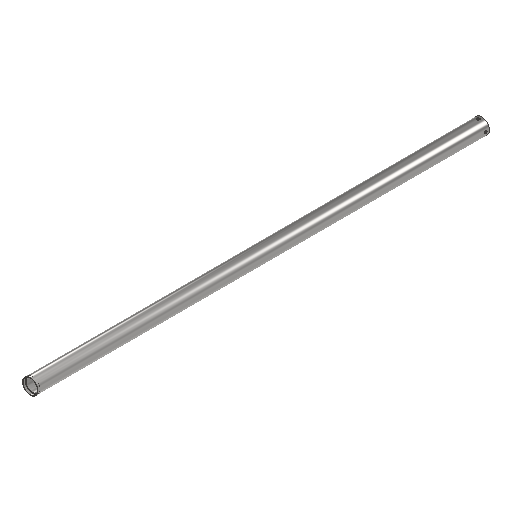
# Autodesk Inventor part: B_probe_pipe_5
Saved by Autodesk Inventor 2026.2 (Build 302298000, 298)
## iProperties
Created: 2026-01-05
Part Number: B_probe_pipe_5
Material: ステンレス鋼 440C
Document SubType Name: Sheet Metal
Designer: 水野 薫哉
Density: 7.75 g/cm^3
Sheet Metal Rule: Default
Appearance: 半つや出し
Author: 水野 薫哉
Autodesk Inventor part; units mm, degrees
ref_plane "XY Plane" through (0, 0, 0) normal (0, 0, 1) x (1, 0, 0)
sketch "スケッチ1" plane through (0, 0, 0) normal (0, 0, 1) x (1, 0, 0)
  circle A0 centre (0, 0) radius 17
  circle A1 centre (0, 0) radius 14.2
  dimension "d0" = 34
  dimension "d1" = 28.4
  constraints: 2 centre point, 2 coincident
  measures "d0" diameter of A0
  measures "d1" diameter of A1
extrude "押し出し1" add sketch "スケッチ1" against normal blind 1000
sketch "スケッチ3" plane through (0, 0, 0) normal (0, 0, 1) x (1, 0, 0)
  circle A0 centre (0, 0) radius 16
  dimension "d8" = 32
  constraints: 1 centre point, 1 coincident
  measures "d8" diameter of A0
extrude "押し出し3" cut sketch "スケッチ3" against normal blind 5
ref_plane "作業平面2" through (17, 0, 0) normal (1, 0, 0) x (0, 1, 0)
ref_plane "作業平面3" through (-17, 0, 0) normal (1, 0, 0) x (0, 1, 0)
ref_plane "作業平面4" through (0, 17, 0) normal (0, 1, 0) x (-1, 0, 0)
ref_plane "作業平面5" through (0, -17, 0) normal (0, 1, 0) x (-1, 0, 0)
sketch "スケッチ8" plane through (17, 0, 0) normal (1, 0, 0) x (0, 1, 0)
  circle A0 centre (0, -992) radius 3.25
  line L0 (-17, -1000) -> (17, -1000) projected
  point P0 (0, 0)
  dimension "d28" = 6.5
  dimension "d29" = 8
  constraints: 1 centre point
  measures "d28" diameter of A0
  measures "d29" distance from line of L0 A0.centre
sketch "スケッチ9" plane through (-17, 0, 0) normal (1, 0, 0) x (0, 1, 0)
  circle A0 centre (0, -992) radius 3.25
  line L0 (-17, -1000) -> (17, -1000) projected
  point P0 (0, 0)
  dimension "d30" = 6.5
  dimension "d31" = 8
  constraints: 1 centre point
  measures "d30" diameter of A0
  measures "d31" distance from line of L0 A0.centre
extrude "押し出し7" cut sketch "スケッチ8" against normal blind 2
extrude "押し出し8" cut sketch "スケッチ9" along normal blind 2
sketch "スケッチ10" plane through (0, 17, 0) normal (0, 1, 0) x (-1, 0, 0)
  circle A0 centre (0, -992) radius 3.25
  line L0 (-17, -1000) -> (17, -1000) projected
  point P0 (0, 0)
  dimension "d36" = 6.5
  dimension "d37" = 8
  constraints: 1 centre point
  measures "d36" diameter of A0
  measures "d37" distance from line of L0 A0.centre
sketch "スケッチ11" plane through (0, -17, 0) normal (0, 1, 0) x (-1, 0, 0)
  circle A0 centre (0, -992) radius 3.25
  line L0 (-17, -1000) -> (17, -1000) projected
  point P0 (0, 0)
  dimension "d38" = 6.5
  dimension "d39" = 8
  constraints: 1 centre point
  measures "d38" diameter of A0
  measures "d39" distance from line of L0 A0.centre
extrude "押し出し9" cut sketch "スケッチ10" against normal blind 2
extrude "押し出し10" cut sketch "スケッチ11" along normal blind 2
sketch "スケッチ12" plane through (0, 0, 0) normal (1, 0, 0) x (0, 1, 0)
  circle A0 centre (0, -992) radius 1.7
  line L0 (-17, -1000) -> (17, -1000) projected
  point P0 (0, 0)
  dimension "d44" = 3.4
  dimension "d45" = 8
  constraints: 1 centre point
  measures "d44" diameter of A0
  measures "d45" distance from line of L0 A0.centre
extrude "押し出し11" cut sketch "スケッチ12" along normal through all both and the other way through all
sketch "スケッチ13" plane through (0, 0, 0) normal (0, 1, 0) x (-1, 0, 0)
  circle A0 centre (0, -992) radius 1.7
  line L0 (-17, -1000) -> (17, -1000) projected
  point P0 (0, 0)
  dimension "d48" = 3.4
  dimension "d49" = 8
  constraints: 1 centre point
  measures "d48" diameter of A0
  measures "d49" distance from line of L0 A0.centre
extrude "押し出し12" cut sketch "スケッチ13" along normal through all both and the other way through all
equation "\"BendRadius\" = Thickness"
equation "\"BendReliefWidth\" = Thickness"
equation "\"BendReliefDepth\" = 0.5 * Thickness"
equation "\"CornerReliefSize\" = 4 * Thickness"
equation "\"MinimumRemnant\" = 2 * Thickness"
equation "\"TransitionRadius\" = BendRadius"
equation "\"JacobiRadiusSize\" = BendRadius"
equation "\"GapSize\" = Thickness"
equation "\"Thickness\" = 3.048"
